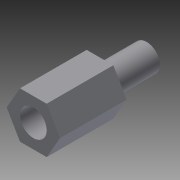
# Autodesk Inventor part: Standoff
Saved by Autodesk Inventor 2015 SP1 (Build 190203100, 203)
## iProperties
Created: 2015-10-19
Part Number: Standoff
Material: Generic
Document SubType Name: Modeling
Designer: Kartikye
Density: 1 g/cm^3
Appearance: Default
Author: Kartikye
Autodesk Inventor part; units mm, degrees
ref_plane "YZ Plane" through (0, 0, 0) normal (1, 0, 0) x (0, 1, 0)
ref_plane "XZ Plane" through (0, 0, 0) normal (0, 1, 0) x (-1, 0, 0)
ref_plane "XY Plane" through (0, 0, 0) normal (0, 0, 1) x (1, 0, 0)
sketch "Sketch1" plane through (0, 0, 0) normal (0, 1, 0) x (-1, 0, 0)
  line L0 (2, 0) -> (1, -1.7321)
  line L1 (1, -1.7321) -> (-1, -1.7321)
  line L2 (-1, -1.7321) -> (-2, 0)
  line L3 (-2, 0) -> (-1, 1.7321)
  line L4 (-1, 1.7321) -> (1, 1.7321)
  line L5 (1, 1.7321) -> (2, 0)
  circle A0 centre (0, 0) radius 1
  constraints: 12 end point, 2 coincident, 1 centre point, 13 other
extrude "Extrusion1" add sketch "Sketch1" along normal blind 5
sketch "Sketch2" plane through (0, 5, 0) normal (0, 1, 0) x (1, 0, 0)
  line L0 (-2, 0) -> (-1, 1.7321)
  line L1 (-1, 1.7321) -> (1, 1.7321)
  line L2 (1, 1.7321) -> (2, 0)
  line L3 (2, 0) -> (1, -1.7321)
  line L4 (1, -1.7321) -> (-1, -1.7321)
  line L5 (-1, -1.7321) -> (-2, 0)
  point P0 (0, 0)
  point P1 (0, 0)
  constraints: 12 end point, 1 coincident, 13 other
extrude "Extrusion2" add sketch "Sketch2" against normal blind 0.1
sketch "Sketch3" plane through (0, 5, 0) normal (0, 1, 0) x (1, 0, 0)
  circle A0 centre (0, 0) radius 1
  dimension "d5" = 2
  constraints: 1 centre point, 1 coincident
  measures "d5" diameter of A0
extrude "Extrusion3" add sketch "Sketch3" along normal blind 3.5
body "Solid1"
